test for drilling generated on Friday first cirlecs then intersect_v1 (Autodesk Fusion 360 design; units mm, degrees)
Autodesk Fusion 360 part; units mm, degrees
sketch "b  stock" plane through (0, 0, 0) normal (0, 0, 1) x (1, 0, 0)
  line L0 (0, 0) -> (304.8, 0)
  line L1 (304.8, 0) -> (304.8, 609.6)
  line L2 (304.8, 609.6) -> (0, 609.6)
  line L3 (0, 609.6) -> (0, 0)
extrude "b  stock body extrude" add sketch "b  stock" along normal blind 3.175 makes body 1
sketch "b  layout" plane through (0, 0, 0) normal (0, 0, 1) x (1, 0, 0)
  line L0 (0, 0) -> (90, 0)
  line L1 (90, 0) -> (90, 85)
  line L2 (90, 85) -> (0, 85)
  line L3 (0, 85) -> (0, 0)
sketch "b top lines" plane through (0, 0, 0) normal (0, 0, 1) x (1, 0, 0)
  line L0 (0, 0) -> (10.15, 0)
  line L1 (10.15, 0) -> (10.15, 3.175)
  line L2 (10.15, 3.175) -> (19.85, 3.175)
  line L3 (19.85, 3.175) -> (19.85, 0)
  line L4 (19.85, 0) -> (30.15, 0)
  line L5 (30.15, 0) -> (30.15, 3.175)
  line L6 (30.15, 3.175) -> (39.85, 3.175)
  line L7 (39.85, 3.175) -> (39.85, 0)
  line L8 (39.85, 0) -> (50.15, 0)
  line L9 (50.15, 0) -> (50.15, 3.175)
  line L10 (50.15, 3.175) -> (59.85, 3.175)
  line L11 (59.85, 3.175) -> (59.85, 0)
  line L12 (59.85, 0) -> (70.15, 0)
  line L13 (70.15, 0) -> (70.15, 3.175)
  line L14 (70.15, 3.175) -> (79.85, 3.175)
  line L15 (79.85, 3.175) -> (79.85, 0)
  line L16 (79.85, 0) -> (90, 0)
  line L17 (90, 0) -> (90, 17.65)
  line L18 (90, 17.65) -> (86.825, 17.65)
  line L19 (86.825, 17.65) -> (86.825, 27.35)
  line L20 (86.825, 27.35) -> (90, 27.35)
  line L21 (90, 27.35) -> (90, 37.65)
  line L22 (90, 37.65) -> (86.825, 37.65)
  line L23 (86.825, 37.65) -> (86.825, 47.35)
  line L24 (86.825, 47.35) -> (90, 47.35)
  line L25 (90, 47.35) -> (90, 57.65)
  line L26 (90, 57.65) -> (86.825, 57.65)
  line L27 (86.825, 57.65) -> (86.825, 67.35)
  line L28 (86.825, 67.35) -> (90, 67.35)
  line L29 (90, 67.35) -> (90, 85)
  line L30 (0, 85) -> (10.15, 85)
  line L31 (10.15, 85) -> (10.15, 81.825)
  line L32 (10.15, 81.825) -> (19.85, 81.825)
  line L33 (19.85, 81.825) -> (19.85, 85)
  line L34 (19.85, 85) -> (30.15, 85)
  line L35 (30.15, 85) -> (30.15, 81.825)
  line L36 (30.15, 81.825) -> (39.85, 81.825)
  line L37 (39.85, 81.825) -> (39.85, 85)
  line L38 (39.85, 85) -> (50.15, 85)
  line L39 (50.15, 85) -> (50.15, 81.825)
  line L40 (50.15, 81.825) -> (59.85, 81.825)
  line L41 (59.85, 81.825) -> (59.85, 85)
  line L42 (59.85, 85) -> (70.15, 85)
  line L43 (70.15, 85) -> (70.15, 81.825)
  line L44 (70.15, 81.825) -> (79.85, 81.825)
  line L45 (79.85, 81.825) -> (79.85, 85)
  line L46 (79.85, 85) -> (90, 85)
  line L47 (0, 0) -> (0, 17.65)
  line L48 (0, 17.65) -> (3.175, 17.65)
  line L49 (3.175, 17.65) -> (3.175, 27.35)
  line L50 (3.175, 27.35) -> (0, 27.35)
  line L51 (0, 27.35) -> (0, 37.65)
  line L52 (0, 37.65) -> (3.175, 37.65)
  line L53 (3.175, 37.65) -> (3.175, 47.35)
  line L54 (3.175, 47.35) -> (0, 47.35)
  line L55 (0, 47.35) -> (0, 57.65)
  line L56 (0, 57.65) -> (3.175, 57.65)
  line L57 (3.175, 57.65) -> (3.175, 67.35)
  line L58 (3.175, 67.35) -> (0, 67.35)
  line L59 (0, 67.35) -> (0, 85)
  dimension "d227" = 10.15
  dimension "d228" = 3.175
  dimension "d229" = 9.7
  dimension "d230" = 3.175
  dimension "d231" = 10.3
  dimension "d232" = 3.175
  dimension "d233" = 9.7
  dimension "d234" = 3.175
  dimension "d235" = 10.3
  dimension "d236" = 3.175
  dimension "d237" = 9.7
  dimension "d238" = 3.175
  dimension "d239" = 10.3
  dimension "d240" = 3.175
  dimension "d241" = 9.7
  dimension "d242" = 3.175
  dimension "d243" = 10.15
  dimension "d252" = 17.65
  dimension "d253" = 3.175
  dimension "d254" = 9.7
  dimension "d255" = 3.175
  dimension "d256" = 10.3
  dimension "d257" = 3.175
  dimension "d258" = 9.7
  dimension "d259" = 3.175
  dimension "d260" = 10.3
  dimension "d261" = 3.175
  dimension "d262" = 9.7
  dimension "d263" = 3.175
  dimension "d264" = 17.65
  dimension "d271" = 10.15
  dimension "d272" = 3.175
  dimension "d273" = 9.7
  dimension "d274" = 3.175
  dimension "d275" = 10.3
  dimension "d276" = 3.175
  dimension "d277" = 9.7
  dimension "d278" = 3.175
  dimension "d279" = 10.3
  dimension "d280" = 3.175
  dimension "d281" = 9.7
  dimension "d282" = 3.175
  dimension "d283" = 10.3
  dimension "d284" = 3.175
  dimension "d285" = 9.7
  dimension "d286" = 3.175
  dimension "d287" = 10.15
  dimension "d296" = 17.65
  dimension "d297" = 3.175
  dimension "d298" = 9.7
  dimension "d299" = 3.175
  dimension "d300" = 10.3
  dimension "d301" = 3.175
  dimension "d302" = 9.7
  dimension "d303" = 3.175
  dimension "d304" = 10.3
  dimension "d305" = 3.175
  dimension "d306" = 9.7
  dimension "d307" = 3.175
  dimension "d308" = 17.65
  constraint horizontal L0
  constraint vertical L1
  constraint horizontal L2
  constraint vertical L3
  constraint horizontal L4
  constraint vertical L5
  constraint horizontal L6
  constraint vertical L7
  constraint horizontal L8
  constraint vertical L9
  constraint horizontal L10
  constraint vertical L11
  constraint horizontal L12
  constraint vertical L13
  constraint horizontal L14
  constraint vertical L15
  constraint horizontal L16
  constraint vertical L17
  constraint horizontal L18
  constraint vertical L19
  constraint horizontal L20
  constraint vertical L21
  constraint horizontal L22
  constraint vertical L23
  constraint horizontal L24
  constraint vertical L25
  constraint horizontal L26
  constraint vertical L27
  constraint horizontal L28
  constraint vertical L29
  constraint horizontal L30
  constraint vertical L31
  constraint horizontal L32
  constraint vertical L33
  constraint horizontal L34
  constraint vertical L35
  constraint horizontal L36
  constraint vertical L37
  constraint horizontal L38
  constraint vertical L39
  constraint horizontal L40
  constraint vertical L41
  constraint horizontal L42
  constraint vertical L43
  constraint horizontal L44
  constraint vertical L45
  constraint horizontal L46
  constraint vertical L47
  constraint horizontal L48
  constraint vertical L49
  constraint horizontal L50
  constraint vertical L51
  constraint horizontal L52
  constraint vertical L53
  constraint horizontal L54
  constraint vertical L55
  constraint horizontal L56
  constraint vertical L57
  constraint horizontal L58
  constraint vertical L59
  measures "d227" distance of L0.start L0.end
  measures "d228" distance of L0.end L1.end
  measures "d229" distance of L1.end L2.end
  measures "d230" distance of L2.end L3.end
  measures "d231" distance of L3.end L4.end
  measures "d232" distance of L4.end L5.end
  measures "d233" distance of L5.end L6.end
  measures "d234" distance of L6.end L7.end
  measures "d235" distance of L7.end L8.end
  measures "d236" distance of L8.end L9.end
  measures "d237" distance of L9.end L10.end
  measures "d238" distance of L10.end L11.end
  measures "d239" distance of L11.end L12.end
  measures "d240" distance of L12.end L13.end
  measures "d241" distance of L13.end L14.end
  measures "d242" distance of L14.end L15.end
  measures "d243" distance of L15.end L16.end
  measures "d252" distance of L16.end L17.end
  measures "d253" distance of L17.end L18.end
  measures "d254" distance of L18.end L19.end
  measures "d255" distance of L19.end L20.end
  measures "d256" distance of L20.end L21.end
  measures "d257" distance of L21.end L22.end
  measures "d258" distance of L22.end L23.end
  measures "d259" distance of L23.end L24.end
  measures "d260" distance of L24.end L25.end
  measures "d261" distance of L25.end L26.end
  measures "d262" distance of L26.end L27.end
  measures "d263" distance of L27.end L28.end
  measures "d264" distance of L28.end L29.end
  measures "d271" distance of L30.start L30.end
  measures "d272" distance of L30.end L31.end
  measures "d273" distance of L31.end L32.end
  measures "d274" distance of L32.end L33.end
  measures "d275" distance of L33.end L34.end
  measures "d276" distance of L34.end L35.end
  measures "d277" distance of L35.end L36.end
  measures "d278" distance of L36.end L37.end
  measures "d279" distance of L37.end L38.end
  measures "d280" distance of L38.end L39.end
  measures "d281" distance of L39.end L40.end
  measures "d282" distance of L40.end L41.end
  measures "d283" distance of L41.end L42.end
  measures "d284" distance of L42.end L43.end
  measures "d285" distance of L43.end L44.end
  measures "d286" distance of L44.end L45.end
  measures "d287" distance of L29.end L45.end
  measures "d296" distance of L0.start L47.end
  measures "d297" distance of L47.end L48.end
  measures "d298" distance of L48.end L49.end
  measures "d299" distance of L49.end L50.end
  measures "d300" distance of L50.end L51.end
  measures "d301" distance of L51.end L52.end
  measures "d302" distance of L52.end L53.end
  measures "d303" distance of L53.end L54.end
  measures "d304" distance of L54.end L55.end
  measures "d305" distance of L55.end L56.end
  measures "d306" distance of L56.end L57.end
  measures "d307" distance of L57.end L58.end
  measures "d308" distance of L30.start L58.end
sketch "b top circles" plane through (0, 0, 0) normal (0, 0, 1) x (1, 0, 0)
  line L0 (0, 0) -> (90, 0)
  line L1 (90, 0) -> (90, 85)
  line L2 (90, 85) -> (0, 85)
  line L3 (0, 85) -> (0, 0)
  circle A0 centre (10.6806, 2.4644) radius 1.005
  circle A1 centre (19.3194, 2.4644) radius 1.005
  circle A2 centre (30.6806, 2.4644) radius 1.005
  circle A3 centre (39.3194, 2.4644) radius 1.005
  circle A4 centre (50.6806, 2.4644) radius 1.005
  circle A5 centre (59.3194, 2.4644) radius 1.005
  circle A6 centre (70.6806, 2.4644) radius 1.005
  circle A7 centre (79.3194, 2.4644) radius 1.005
  circle A8 centre (87.5356, 18.1806) radius 1.005
  circle A9 centre (87.5356, 26.8194) radius 1.005
  circle A10 centre (87.5356, 38.1806) radius 1.005
  circle A11 centre (87.5356, 46.8194) radius 1.005
  circle A12 centre (87.5356, 58.1806) radius 1.005
  circle A13 centre (87.5356, 66.8194) radius 1.005
  circle A14 centre (10.6806, 82.5356) radius 1.005
  circle A15 centre (19.3194, 82.5356) radius 1.005
  circle A16 centre (30.6806, 82.5356) radius 1.005
  circle A17 centre (39.3194, 82.5356) radius 1.005
  circle A18 centre (50.6806, 82.5356) radius 1.005
  circle A19 centre (59.3194, 82.5356) radius 1.005
  circle A20 centre (70.6806, 82.5356) radius 1.005
  circle A21 centre (79.3194, 82.5356) radius 1.005
  circle A22 centre (2.4644, 18.1806) radius 1.005
  circle A23 centre (2.4644, 26.8194) radius 1.005
  circle A24 centre (2.4644, 38.1806) radius 1.005
  circle A25 centre (2.4644, 46.8194) radius 1.005
  circle A26 centre (2.4644, 58.1806) radius 1.005
  circle A27 centre (2.4644, 66.8194) radius 1.005
  dimension "d244" = 2.01
  dimension "d245" = 2.01
  dimension "d246" = 2.01
  dimension "d247" = 2.01
  dimension "d248" = 2.01
  dimension "d249" = 2.01
  dimension "d250" = 2.01
  dimension "d251" = 2.01
  dimension "d265" = 2.01
  dimension "d266" = 2.01
  dimension "d267" = 2.01
  dimension "d268" = 2.01
  dimension "d269" = 2.01
  dimension "d270" = 2.01
  dimension "d288" = 2.01
  dimension "d289" = 2.01
  dimension "d290" = 2.01
  dimension "d291" = 2.01
  dimension "d292" = 2.01
  dimension "d293" = 2.01
  dimension "d294" = 2.01
  dimension "d295" = 2.01
  dimension "d309" = 2.01
  dimension "d310" = 2.01
  dimension "d311" = 2.01
  dimension "d312" = 2.01
  dimension "d313" = 2.01
  dimension "d314" = 2.01
  measures "d244" diameter of A0
  measures "d245" diameter of A1
  measures "d246" diameter of A2
  measures "d247" diameter of A3
  measures "d248" diameter of A4
  measures "d249" diameter of A5
  measures "d250" diameter of A6
  measures "d251" diameter of A7
  measures "d265" diameter of A8
  measures "d266" diameter of A9
  measures "d267" diameter of A10
  measures "d268" diameter of A11
  measures "d269" diameter of A12
  measures "d270" diameter of A13
  measures "d288" diameter of A14
  measures "d289" diameter of A15
  measures "d290" diameter of A16
  measures "d291" diameter of A17
  measures "d292" diameter of A18
  measures "d293" diameter of A19
  measures "d294" diameter of A20
  measures "d295" diameter of A21
  measures "d309" diameter of A22
  measures "d310" diameter of A23
  measures "d311" diameter of A24
  measures "d312" diameter of A25
  measures "d313" diameter of A26
  measures "d314" diameter of A27
extrude "b top lines body extrude" add sketch "b top lines" along normal blind 3.175 separate body makes body 2
extrude "b top circles extrude" add sketch "b top circles" along normal blind 3.175 separate body makes body 3
combine "b top lines final combine feature" operation intersect target body 2 tool bodies 3
equation "Version_info = 0 mm" comment "1.0.0 LENGTH 90 DEPTH 85 HEIGHT 50 THICKNESS 3.175 TOOL_DIAMETER 2.01 TOOTH_WIDTH 10 KERF -0.15 DELTA_FROM_BOTTOM -0.1 STOCK_X_DIMENSION 304.8 STOCK_Y_DIMENSION 609.6 COMPONENT   REPEATS_L_TMP -1 CREATE_COMPONENTS False CREATE_BODIES 1 CREATE_EMPTY_CONTENTS False CREATE_CONSTRAINTS True CLEAR_PREVIOUSLY_GENERATED_ITEMS True JUST_CLEAR_PREVIOUSLY_GENERATED_ITEMS False CREATE_MANUFACTURING False CREATE_LAYOUT True DEBUG_JUST_ONE_PART True DEBUG True"
equation "Length = 90.0 mm" comment "Length (mm)"
equation "Depth = 85.0 mm" comment "Depth (mm)"
equation "Height = 50.0 mm" comment "Height (mm)"
equation "Thickness = 3.175 mm" comment "Thickness (mm)"
equation "Tool_diameter = 2.01 mm" comment "Tool Diameter (mm)"
equation "Tooth_width = 10.0 mm" comment "Target Tooth Width (mm)"
equation "Kerf = -0.15 mm" comment "Kerf (mm)- can be negative"
equation "Delta_from_bottom = 0.0 mm" comment "Additional fine adjustment of bone centers from bottom of holes(mm)- positive makes smaller bottom indents"
equation "Stock_x_dimension = 304.8 mm" comment "Stock X Dimension"
equation "Stock_y_dimension = 609.6 mm" comment "Stock Y Dimension"
equation "Repeats_l_tmp = -1.0 mm" comment "temp hidden"
equation "d228 = Thickness"
equation "d230 = Thickness"
equation "d232 = Thickness"
equation "d234 = Thickness"
equation "d236 = Thickness"
equation "d238 = Thickness"
equation "d240 = Thickness"
equation "d242 = Thickness"
equation "d244 = Tool_diameter"
equation "d245 = Tool_diameter"
equation "d246 = Tool_diameter"
equation "d247 = Tool_diameter"
equation "d248 = Tool_diameter"
equation "d249 = Tool_diameter"
equation "d250 = Tool_diameter"
equation "d251 = Tool_diameter"
equation "d253 = Thickness"
equation "d255 = Thickness"
equation "d257 = Thickness"
equation "d259 = Thickness"
equation "d261 = Thickness"
equation "d263 = Thickness"
equation "d265 = Tool_diameter"
equation "d266 = Tool_diameter"
equation "d267 = Tool_diameter"
equation "d268 = Tool_diameter"
equation "d269 = Tool_diameter"
equation "d270 = Tool_diameter"
equation "d272 = Thickness"
equation "d274 = Thickness"
equation "d276 = Thickness"
equation "d278 = Thickness"
equation "d280 = Thickness"
equation "d282 = Thickness"
equation "d284 = Thickness"
equation "d286 = Thickness"
equation "d288 = Tool_diameter"
equation "d289 = Tool_diameter"
equation "d290 = Tool_diameter"
equation "d291 = Tool_diameter"
equation "d292 = Tool_diameter"
equation "d293 = Tool_diameter"
equation "d294 = Tool_diameter"
equation "d295 = Tool_diameter"
equation "d297 = Thickness"
equation "d299 = Thickness"
equation "d301 = Thickness"
equation "d303 = Thickness"
equation "d305 = Thickness"
equation "d307 = Thickness"
equation "d309 = Tool_diameter"
equation "d310 = Tool_diameter"
equation "d311 = Tool_diameter"
equation "d312 = Tool_diameter"
equation "d313 = Tool_diameter"
equation "d314 = Tool_diameter"
named bodies: "b  stock body", "b top  body", "b top circles cheese body"
